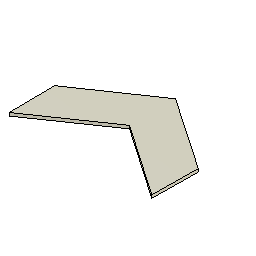
Adaptação_barco_frente v2 (Autodesk Fusion 360 design; units mm, degrees)
Autodesk Fusion 360 part; units mm, degrees
sketch "Esboço1" plane through (0, 0, 0) normal (0, 0, 1) x (1, 0, 0)
  line L0 (0, 0) -> (88, 0)
  line L1 (-2.5, 203) -> (0, 0)
  line L2 (90.5, 203) -> (88, 0)
  line L3 (44, 235) -> (90.5, 203)
  line L4 (44, 235) -> (-2.5, 203)
  line L5 (88.487, 201.9575) -> (86.0245, 2)
  line L6 (1.9755, 2) -> (86.0245, 2)
  line L7 (-0.487, 201.9575) -> (1.9755, 2)
  line L8 (44, 232.5722) -> (-0.487, 201.9575)
  line L9 (44, 232.5722) -> (88.487, 201.9575)
  dimension "d1" = 88
  dimension "d7" = -2
  constraint coincident L0.start L1.end
  constraint horizontal L0
  measures "d1" distance of L0.start L0.end
sketch "Esboço2" plane through (0, 0, 5) normal (0, 0, 1) x (-1, 0, 0)
  line L0 (-1.9755, -2) -> (0.487, -201.9575)
  line L1 (0.487, -201.9575) -> (-44, -232.5722)
  line L2 (-44, -232.5722) -> (-88.487, -201.9575)
  line L3 (-88.487, -201.9575) -> (-86.0245, -2)
  line L4 (-86.0245, -2) -> (-1.9755, -2)
  line L5 (-90.5, -203) -> (-44, -235)
  line L6 (-44, -235) -> (2.5, -203)
  line L7 (2.5, -203) -> (0, 0)
  line L8 (0, 0) -> (-88, 0)
  line L9 (-88, 0) -> (-90.5, -203)
  line L10 (-44, -228.9304) -> (-85.4675, -200.3937)
  line L11 (-85.4675, -200.3937) -> (-83.0612, -5)
  line L12 (-83.0612, -5) -> (-4.9388, -5)
  line L13 (-4.9388, -5) -> (-2.5325, -200.3937)
  line L14 (-2.5325, -200.3937) -> (-44, -228.9304)
  dimension "d10" = 3
sketch "Esboço3" plane through (0, 0, 5) normal (0, 0, 1) x (-1, 0, 0)
  line L0 (-4.9388, -5) -> (-2.5325, -200.3937)
  line L1 (-2.5325, -200.3937) -> (-44, -228.9304)
  line L2 (-44, -228.9304) -> (-85.4675, -200.3937)
  line L3 (-85.4675, -200.3937) -> (-83.0612, -5)
  line L4 (-83.0612, -5) -> (-4.9388, -5)
  line L5 (-4.0422, -199.6117) -> (-44, -227.1096)
  line L6 (-44, -227.1096) -> (-83.9578, -199.6117)
  line L7 (-83.9578, -199.6117) -> (-81.5796, -6.5)
  line L8 (-81.5796, -6.5) -> (-6.4204, -6.5)
  line L9 (-6.4204, -6.5) -> (-4.0422, -199.6117)
  line L10 (-86.0245, -2) -> (-88.487, -201.9575)
  line L11 (-88.487, -201.9575) -> (-44, -232.5722)
  line L12 (-44, -232.5722) -> (0.487, -201.9575)
  line L13 (0.487, -201.9575) -> (-1.9755, -2)
  line L14 (-1.9755, -2) -> (-86.0245, -2)
  dimension "d13" = 1.5
sketch "Esboço4" plane through (0, 0, 5) normal (0, 0, 1) x (-1, 0, 0)
  line L0 (-81.5796, -6.5) -> (-6.4204, -6.5)
  line L1 (-6.4204, -6.5) -> (-4.0422, -199.6117)
  line L2 (-4.0422, -199.6117) -> (-44, -227.1096)
  line L3 (-44, -227.1096) -> (-83.9578, -199.6117)
  line L4 (-83.9578, -199.6117) -> (-81.5796, -6.5)
  line L5 (-44, -233.1791) -> (0.9903, -202.2181)
  line L6 (0.9903, -202.2181) -> (-1.4816, -1.5)
  line L7 (-1.4816, -1.5) -> (-86.5184, -1.5)
  line L8 (-86.5184, -1.5) -> (-88.9903, -202.2181)
  line L9 (-88.9903, -202.2181) -> (-44, -233.1791)
  line L10 (-83.0612, -5) -> (-85.4675, -200.3937)
  line L11 (-85.4675, -200.3937) -> (-44, -228.9304)
  line L12 (-44, -228.9304) -> (-2.5325, -200.3937)
  line L13 (-2.5325, -200.3937) -> (-4.9388, -5)
  line L14 (-4.9388, -5) -> (-83.0612, -5)
sketch "Esboço5" plane through (86.4868, -1.0651, 0) normal (-0.999924, 0.012314, 0) x (-0.012314, -0.999924, 0)
  line L0 (-2.5653, 5) -> (-2.5653, 65)
  line L1 (-2.5653, 65) -> (-203.2986, 65)
  line L2 (-203.2986, 65) -> (-203.2986, 5)
  line L3 (-2.5653, 65) -> (-2.5653, 63)
  line L4 (-2.5653, 63) -> (-10.5653, 63)
  line L5 (-10.5653, 63) -> (-10.5653, 60)
  line L6 (-10.5653, 60) -> (-2.5653, 60)
  line L7 (-203.2986, 5) -> (-2.5653, 5)
  dimension "d19" = 2
  dimension "d20" = 8
  dimension "d21" = 3
  constraint coincident L0.end L1.start
  constraint perpendicular L1 L3
  constraint perpendicular L3 L4
  constraint perpendicular L4 L5
  constraint coincident L0 L6.end
  constraint perpendicular L0 L6
  measures "d19" distance of L0.end L3.end
  measures "d20" distance of L3.end L4.end
  measures "d21" distance of L4.end L5.end
sketch "Esboço6" plane through (0, 0, 63) normal (0, 0, 1) x (-1, 0, 0)
  line L0 (-86.6169, -9.4994) -> (-78.6175, -9.5979)
  line L1 (-78.6175, -9.5979) -> (-78.519, -1.5985)
  line L2 (-78.519, -1.5985) -> (-86.5184, -1.5)
  line L3 (-78.519, -1.5985) -> (-86.6169, -9.4994)
  line L4 (-86.5184, -1.5) -> (-86.6169, -9.4994)
  constraint coincident L1.end L2.start
  constraint coincident L0.start L3.end
sketch "Esboço7" plane through (0, 0, 63) normal (0, 0, 1) x (-1, 0, 0)
  line L0 (-86.6169, -9.4994) -> (-78.519, -1.5985)
  line L1 (-78.519, -1.5985) -> (-86.5184, -1.5)
  circle A0 centre (-84.5431, -3.5245) radius 1
  line L2 (-86.5184, -1.5) -> (-86.6169, -9.4994)
  dimension "d26" = 2
  measures "d26" diameter of A0
sketch "Esboço8" plane through (1.4999, 0.0185, 0) normal (0.999924, 0.012314, 0) x (-0.012314, 0.999924, 0)
  line L0 (202.215, 5) -> (202.215, 65)
  line L1 (202.215, 65) -> (1.4816, 65)
  line L2 (1.4816, 65) -> (1.4816, 5)
  line L3 (1.4816, 65) -> (1.4816, 63)
  line L4 (1.4816, 63) -> (9.4816, 63)
  line L5 (9.4816, 63) -> (9.4816, 60)
  line L6 (9.4816, 60) -> (1.4816, 60)
  line L7 (1.4816, 5) -> (202.215, 5)
  dimension "d29" = 2
  dimension "d30" = 8
  constraint coincident L1.end L2.start
  constraint perpendicular L1 L3
  constraint perpendicular L3 L4
  constraint perpendicular L4 L5
  constraint coincident L2 L6.end
  constraint perpendicular L2 L6
  measures "d29" distance of L1.end L3.end
  measures "d30" distance of L3.end L4.end
sketch "Esboço9" plane through (0, 0, 63) normal (0, 0, 1) x (-1, 0, 0)
  line L0 (-1.4816, -1.5) -> (-9.481, -1.5985)
  line L1 (-9.481, -1.5985) -> (-9.3825, -9.5979)
  line L2 (-9.3825, -9.5979) -> (-1.3831, -9.4994)
  line L3 (-9.481, -1.5985) -> (-1.3831, -9.4994)
  line L4 (-1.3831, -9.4994) -> (-1.4816, -1.5)
  constraint coincident L0.end L1.start
  constraint coincident L2.end L3.end
sketch "Esboço10" plane through (0, 0, 63) normal (0, 0, 1) x (-1, 0, 0)
  line L0 (-9.481, -1.5985) -> (-1.3831, -9.4994)
  line L1 (-1.4816, -1.5) -> (-9.481, -1.5985)
  circle A0 centre (-3.4569, -3.5245) radius 1
  line L2 (-1.3831, -9.4994) -> (-1.4816, -1.5)
  dimension "d35" = 2
  measures "d35" diameter of A0
sketch "Esboço11" plane through (-94.7554, 137.6915, 0) normal (0.566905, -0.823783, 0) x (0.823783, 0.566905, 0)
  line L0 (168.4368, 5) -> (168.4368, 65)
  line L1 (168.4368, 65) -> (113.8226, 65)
  line L2 (113.8226, 65) -> (113.8226, 5)
  line L3 (113.8226, 5) -> (168.4368, 5)
sketch "Esboço12" plane through (0, 0, 0) normal (0, 0, 1) x (1, 0, 0)
ref_plane "Plano de trabalho2" through (0, 0, 60) normal (0, 0, 1) x (1, 0, 0)
sketch "Esboço13" plane through (0, 0, 60) normal (0, 0, 1) x (1, 0, 0)
  line L0 (44, 229.2) -> (38, 229.2)
  line L1 (44, 229.2) -> (49.6973, 229.2)
  line L2 (38, 229.2) -> (44, 233.5)
  line L3 (44, 233.5) -> (49.6973, 229.2)
sketch "Esboço14" plane through (0, 0, 63) normal (0, 0, 1) x (-1, 0, 0)
  line L0 (-38, -229.2) -> (-49.6973, -229.2)
  line L1 (-49.6973, -229.2) -> (-44, -233.5)
  circle A0 centre (-43.9788, -231.1896) radius 1
  line L2 (-44, -233.5) -> (-38, -229.2)
  dimension "d48" = 2
  measures "d48" diameter of A0
sketch "Esboço15" plane through (0, 0, 65) normal (0, 0, 1) x (-1, 0, 0)
  line L0 (-44, -233.1791) -> (-88.9903, -202.2181)
  line L1 (-88.9903, -202.2181) -> (-86.5184, -1.5)
  line L2 (-86.5184, -1.5) -> (-1.4816, -1.5)
  line L3 (-1.4816, -1.5) -> (0.9903, -202.2181)
  line L4 (0.9903, -202.2181) -> (-44, -233.1791)
  line L5 (-88, 0) -> (-90.5, -203)
  line L6 (-90.5, -203) -> (-44, -235)
  line L7 (-44, -235) -> (2.5, -203)
  line L8 (2.5, -203) -> (0, 0)
  line L9 (0, 0) -> (-88, 0)
  line L10 (-196.5184, -1.5) -> (-111.4816, -1.5)
  line L11 (-198.9903, -202.2181) -> (-196.5184, -1.5)
  line L12 (-111.4816, -1.5) -> (-109.0097, -202.2181)
  line L13 (168.4368, 65) -> (113.8226, 65)
  line L14 (168.4368, 65) -> (113.8226, 65)
  line L15 (168.4368, 65) -> (113.8226, 65)
  line L16 (-154, -233.1791) -> (-198.9903, -202.2181)
  line L17 (-109.0097, -202.2181) -> (-154, -233.1791)
sketch "Esboço16" plane through (0, 0, 63) normal (0, 0, 1) x (-1, 0, 0)
  line L0 (-38, -229.2) -> (-49.6973, -229.2)
  line L1 (-49.6973, -229.2) -> (-44, -233.5)
  line L2 (-44, -233.5) -> (-38, -229.2)
sketch "Esboço17" plane through (0, 0, 67) normal (0, 0, 1) x (-1, 0, 0)
  line L0 (-109.0097, -202.2181) -> (-111.4816, -1.5)
  line L1 (-111.4816, -1.5) -> (-196.5184, -1.5)
  line L2 (-196.5184, -1.5) -> (-198.9903, -202.2181)
  line L3 (-198.9903, -202.2181) -> (-154, -233.1791)
  line L4 (-154, -233.1791) -> (-109.0097, -202.2181)
  circle A0 centre (-154, -231.1891) radius 1
  dimension "d55" = 1.99
  dimension "d56" = 2
  measures "d55" distance of L3.end A0.centre
  measures "d56" diameter of A0
sketch "Esboço18" plane through (0, 0, 63) normal (0, 0, 1) x (-1, 0, 0)
  circle A0 centre (-84.5431, -3.5245) radius 1
  line L0 (-86.6169, -9.4994) -> (-78.519, -1.5985)
  line L1 (-78.519, -1.5985) -> (-86.5184, -1.5)
  line L2 (-86.5184, -1.5) -> (-86.6169, -9.4994)
sketch "Esboço19" plane through (0, 0, 67) normal (0, 0, 1) x (-1, 0, 0)
  circle A0 centre (-154, -231.1891) radius 1
  line L0 (-109.0097, -202.2181) -> (-111.4816, -1.5)
  line L1 (-111.4816, -1.5) -> (-196.5184, -1.5)
  line L2 (-196.5184, -1.5) -> (-198.9903, -202.2181)
  line L3 (-198.9903, -202.2181) -> (-154, -233.1791)
  line L4 (-154, -233.1791) -> (-109.0097, -202.2181)
  circle A1 centre (-194.2131, -3.138) radius 1
  circle A2 centre (-113.2857, -2.8975) radius 1
  dimension "d59" = 2.828
  dimension "d60" = 2
  dimension "d61" = 2.282
  dimension "d62" = 2
  measures "d59" distance of L1.end A1.centre
  measures "d60" diameter of A1
  measures "d61" distance of L0.end A2.centre
  measures "d62" diameter of A2
sketch "Esboço20" plane through (0, 0, 65) normal (0, 0, 1) x (-1, 0, 0)
  line L0 (-44, -233.1791) -> (-88.9903, -202.2181)
  line L1 (-88.9903, -202.2181) -> (-86.5184, -1.5)
  line L2 (-86.5184, -1.5) -> (-1.4816, -1.5)
  line L3 (-1.4816, -1.5) -> (0.9903, -202.2181)
  line L4 (0.9903, -202.2181) -> (-44, -233.1791)
  line L5 (-88, 0) -> (-90.5, -203)
  line L6 (-90.5, -203) -> (-44, -235)
  line L7 (-44, -235) -> (2.5, -203)
  line L8 (2.5, -203) -> (0, 0)
  line L9 (0, 0) -> (-88, 0)
  line L10 (-44, -235) -> (2.5, -203)
  line L11 (-90.5, -203) -> (-90.8694, -232.9977)
  line L12 (-90.8694, -232.9977) -> (-44, -265)
  line L13 (2.5, -203) -> (2.8694, -232.9977)
  line L14 (2.8694, -232.9977) -> (-44, -265)
  line L15 (-90.5, -203) -> (-44, -235)
  dimension "d65" = 30
  dimension "d66" = 30
  dimension "d67" = 30
  constraint coincident L6.end L7.start
  constraint coincident L7.end L8.start
  constraint coincident L5.end L6.start
  constraint parallel L5 L11
  constraint parallel L8 L13
  measures "d65" distance of L6.end L12.end
  measures "d66" distance of L5.end L11.end
  measures "d67" distance of L7.end L13.end
extrude "Extrusão17" add sketch "Esboço20" against normal blind 2 contours L6 L7 L10 L11 L12 L13 L14 L15
